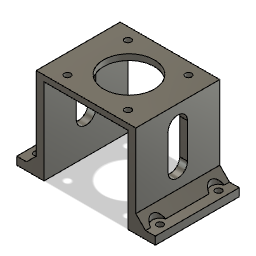
motor_support (Autodesk Fusion 360 design; units mm, degrees)
Autodesk Fusion 360 part; units mm, degrees
note: some values were not read from the file. Set by a fixed rule: which sketch regions a step uses.
sketch "Sketch1" plane through (0, 0, 0) normal (0, 0, 1) x (1, 0, 0)
  line L0 (-35.5, 0) -> (-21.5, 0)
  line L1 (-21.5, 0) -> (-21.5, 44)
  line L2 (-21.5, 44) -> (21.5, 44)
  line L3 (21.5, 44) -> (21.5, 0)
  line L4 (21.5, 0) -> (35.5, 0)
  line L5 (35.5, 0) -> (35.5, 4)
  line L6 (35.5, 4) -> (25.5, 4)
  line L7 (25.5, 4) -> (25.5, 47)
  line L8 (25.5, 47) -> (-25.5, 47)
  line L9 (-25.5, 47) -> (-25.5, 4)
  line L10 (-25.5, 4) -> (-35.5, 4)
  line L11 (-35.5, 4) -> (-35.5, 0)
  dimension "d1" = 43
  dimension "d2" = 21.5
  dimension "d3" = 4
  dimension "d4" = 4
  dimension "d5" = 3
  dimension "d6" = 4
  dimension "d7" = 4
  dimension "d8" = 10
  dimension "d9" = 10
  dimension "d42" = 44
  dimension "d43" = 44
  constraint horizontal L0
  constraint perpendicular L0 L1
  constraint perpendicular L1 L2
  constraint perpendicular L2 L3
  constraint perpendicular L1 L4
  constraint perpendicular L4 L5
  constraint perpendicular L5 L6
  constraint perpendicular L6 L7
  constraint perpendicular L5 L8
  constraint perpendicular L8 L9
  constraint perpendicular L9 L10
  measures "d1" distance of L1.end L2.end
  measures "d2" distance of origin L3
  measures "d3" distance of L3 L7
  measures "d4" distance of L1 L9
  measures "d5" distance of L2 L8
  measures "d6" distance of L4.end L5.end
  measures "d7" distance of L0 L10
  measures "d8" distance of L5.end L6.end
  measures "d9" distance of L9.end L10.end
  measures "d42" distance of L2.end L3.end
  measures "d43" distance of L0.end L1.end
extrude "Extrude1" add sketch "Sketch1" along normal blind 43
sketch "Sketch3" plane through (0, 44, 0) normal (0, -1, 0) x (1, 0, 0)
  line L0 (-21.5, 0) -> (21.5, 0)
  line L1 (21.5, 0) -> (21.5, 43)
  line L2 (21.5, 43) -> (-21.5, 43)
  line L3 (-21.5, 43) -> (-21.5, 0)
  circle A0 centre (-15.5, 6) radius 1.65
  circle A1 centre (15.5, 6) radius 1.65
  circle A2 centre (-15.5, 37) radius 1.65
  circle A3 centre (15.5, 37) radius 1.65
  dimension "d14" = 3.3
  dimension "d15" = 6
  dimension "d16" = 6
  dimension "d19" = 31
  dimension "d20" = 31
  measures "d14" diameter of A0
  measures "d15" distance of L0 A0.centre
  measures "d16" distance of L3 A0.centre
extrude "Extrude2" cut sketch "Sketch3" against normal up to surface (3 mm away) contours A0 | A1 | A2 | A3
chamfer "Chamfer1" distance 5 angle 45 2 edges at (25.5, 4, 21.5) (-25.5, 4, 21.5)
sketch "Sketch5" plane through (0, 44, 0) normal (0, -1, 0) x (1, 0, 0)
  circle A0 centre (15.5, 37) radius 1.65
  circle A1 centre (15.5, 6) radius 1.65
  circle A2 centre (-15.5, 37) radius 1.65
  circle A3 centre (-15.5, 6) radius 1.65
  line L0 (-21.5, 0) -> (21.5, 0)
  line L1 (21.5, 0) -> (21.5, 43)
  line L2 (21.5, 43) -> (-21.5, 43)
  line L3 (-21.5, 43) -> (-21.5, 0)
  circle A4 centre (0, 21) radius 13
  dimension "d25" = 26
  dimension "d26" = 21.5
  measures "d25" diameter of A4
  measures "d26" distance of L3 A4.centre
extrude "Extrude3" cut sketch "Sketch5" against normal up to surface (3 mm away) contours A4
sketch "Sketch6" plane through (0, 0, 0) normal (0, -1, 0) x (1, 0, 0)
  line L0 (21.5, 0) -> (35.5, 0)
  line L1 (35.5, 0) -> (35.5, 43)
  line L2 (35.5, 43) -> (21.5, 43)
  line L3 (21.5, 43) -> (21.5, 0)
  circle A0 centre (31.5, 36.6) radius 1.65
  circle A1 centre (-31.5, 36.6) radius 1.65
  line L4 (-21.5, 0) -> (-21.5, 43)
  line L5 (-35.5, 43) -> (-21.5, 43)
  circle A2 centre (31.5, 6.6) radius 1.65
  circle A3 centre (-31.5, 6.6) radius 1.65
  dimension "d29" = 3.3
  dimension "d30" = 10
  dimension "d31" = 3.3
  dimension "d32" = 10
  dimension "d33" = 6.4
  dimension "d34" = 6.4
  dimension "d37" = 0
  dimension "d38" = -30
  measures "d29" diameter of A0
  measures "d30" distance of L3 A0.centre
  measures "d31" diameter of A1
  measures "d32" distance of A1.centre L4
  measures "d33" distance of L2 A0.centre
  measures "d34" distance of A1.centre L5
extrude "Extrude4" cut sketch "Sketch6" against normal blind 10 contours A0 | A1 | A2 | A3
sketch "Sketch7" plane through (0, 4, 0) normal (0, 1, 0) x (-1, 0, 0)
  arc A0 (-30.5, 7.9124) -> (-30.5, 5.2876) centre (-31.5, 6.6) ccw
  line L0 (-30.5, 7.9124) -> (-30.5, 35.2876)
  arc A1 (-30.5, 37.9124) -> (-30.5, 35.2876) centre (-31.5, 36.6) ccw
  line L1 (-30.5, 37.9124) -> (-30.5, 43)
  line L2 (-30.5, 43) -> (-35.5, 43)
  line L3 (-35.5, 43) -> (-35.5, 0)
  line L4 (-35.5, 0) -> (-30.5, 0)
  line L5 (-30.5, 0) -> (-30.5, 5.2876)
  circle A2 centre (-31.5, 6.6) radius 4
  circle A3 centre (31.5, 6.6) radius 4
  circle A4 centre (-31.5, 36.6) radius 4
  circle A5 centre (31.5, 36.6) radius 4
  dimension "d44" = 8
  dimension "d47" = 63
  dimension "d48" = 30
  constraint concentric A0 A2
  measures "d44" diameter of A2
extrude "Extrude5" cut sketch "Sketch7" along normal blind 4 contours A0 L0 L5 A2 | A0 L0 L5 A2 | L0 A1 L1 A4 | L0 A1 L1 A4 | A3 | A5
sketch "Sketch8" plane through (25.5, 0, 0) normal (1, 0, 0) x (0, 0, -1)
  line L0 (-43, 9) -> (0, 9)
  line L1 (0, 9) -> (0, 47)
  line L2 (0, 47) -> (-43, 47)
  line L3 (-43, 47) -> (-43, 9)
  line L4 (-26.5, 37) -> (-26.5, 19)
  arc A0 (-26.5, 19) -> (-16.5, 19) centre (-21.5, 19) ccw
  line L5 (-16.5, 19) -> (-16.5, 37)
  arc A1 (-16.5, 37) -> (-26.5, 37) centre (-21.5, 37) ccw
  line L6 (-21.5, 37) -> (-21.5, 19) construction
  dimension "d51" = 18
  dimension "d52" = 10
  dimension "d53" = 21.5
  constraint tangent L4 A0
  constraint tangent A0 L5
  constraint parallel L4 L5
  constraint tangent L5 A1
  constraint tangent L4 A1
  constraint vertical L6
  measures "d51" distance of A1.centre A0.centre
  measures "d52" distance of L2 A1.centre
  measures "d53" distance of L1 A1.centre
extrude "Extrude6" cut sketch "Sketch8" against normal up to surface (51 mm away) contours L4 A0 L5 A1
equation "d1 = size"
equation "d2 = d1 / 2"
equation "d4 = d3"
equation "d7 = d6"
equation "d9 = d8"
equation "d10 = size"
equation "size = 43 mm"
equation "spacing = 31 mm"
equation "d15 = ( size - spacing ) / 2"
equation "d16 = d15"
equation "d26 = size / 2"
equation "d32 = d30"
equation "d34 = d33"
equation "d38 = -( size - 13 mm )"
equation "d43 = d42"
equation "d53 = ( 43 / 2 ) * 1 mm"
